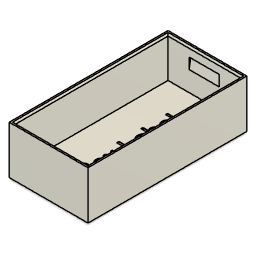
Box Template (Autodesk Fusion 360 design; units mm, degrees)
Autodesk Fusion 360 part; units mm, degrees
sketch "Base" plane through (0, 0, 0) normal (0, 1, 0) x (1, 0, 0)
  line L0 (0, 0) -> (50.8, 0) construction
  line L1 (50.8, 0) -> (50.8, 101.6) construction
  line L2 (50.8, 101.6) -> (0, 101.6) construction
  line L3 (0, 101.6) -> (0, 0) construction
  circle A0 centre (25.4, 25.4) radius 5.9055
  circle A1 centre (25.4, 76.2) radius 5.9055
  line L4 (50.419, 0.381) -> (50.419, 101.219)
  line L5 (50.419, 101.219) -> (0.381, 101.219)
  line L6 (0.381, 101.219) -> (0.381, 0.381)
  line L7 (0.381, 0.381) -> (50.419, 0.381)
  dimension "d1" = 50.8
  dimension "d2" = 101.6
  dimension "d3" = 11.811
  dimension "d5" = 25.4
  dimension "d6" = 25.4
  dimension "d9" = 50.8
  dimension "d10" = 50.8
  constraint horizontal L0
  constraint vertical L1
  constraint horizontal L2
  constraint vertical L3
  constraint coincident L0.start L3.end
  measures "d1" distance of L0.start L0.end
  measures "d2" distance of L0.start L2.end
  measures "d3" diameter of A0
  measures "d5" distance of L0 A0.centre
  measures "d6" distance of L3 A0.centre
extrude "Extrude1" add sketch "Base" along normal blind 6.35 contours A0 | A1 | L4 L5 L6 L7 makes body 1
extrude "Extrude2" cut sketch "Base" along normal blind 5.334 contours A0 bodies 1
chamfer "Chamfer2" distance 1.27 angle 45 1 edges at (19.8941, 0, -23.2645) on bodies 1
pattern_linear "R-Pattern1" count 1 spacing 50.8 along (1, 0, 0) count 2 spacing 50.8 along (0, 0, -1) of "Extrude2", "Chamfer2"
chamfer "Chamfer1" distance 1.27 angle 45 4 edges at (50.419, 0, -50.8) (25.4, 0, -0.381) (0.381, 0, -50.8) (25.4, 0, -101.219) on bodies 1
sketch "Bottom" plane through (0, 6.35, 0) normal (0, 1, 0) x (-1, 0, 0)
  line L0 (-50.419, -101.219) -> (-0.381, -101.219)
  line L1 (-50.419, -0.381) -> (-50.419, -101.219)
  line L2 (-0.381, -0.381) -> (-50.419, -0.381)
  line L3 (-0.381, -101.219) -> (-0.381, -0.381)
  line L4 (-2.413, -2.413) -> (-48.387, -2.413)
  line L5 (-48.387, -2.413) -> (-48.387, -99.187)
  line L6 (-48.387, -99.187) -> (-2.413, -99.187)
  line L7 (-2.413, -99.187) -> (-2.413, -2.413)
  line L8 (-48.387, -2.413) -> (-48.387, -99.187) construction
  line L9 (-48.387, -99.187) -> (-2.413, -99.187) construction
  line L10 (-2.413, -99.187) -> (-2.413, -2.413) construction
  line L11 (-2.413, -2.413) -> (-48.387, -2.413) construction
  dimension "d32" = 2.032
  dimension "d33" = 2.032
  dimension "d34" = 2.032
  dimension "d35" = 2.032
  dimension "d54" = 10.0076
  text T0 "Box Label" font "Arial" height 10.0076 align centre middle in box 96.774 x 45.974 at (-48.387, -2.413) x (0, -1) y (1, 0) spacing 1
  constraint horizontal L6
  constraint horizontal L4
  constraint vertical L5
  constraint vertical L7
  constraint coincident L5.end
  constraint coincident L6.end
  constraint coincident L4.end
  measures "d32" distance of L1 L5
  measures "d33" distance of L3 L7
  measures "d34" distance of L2 L4
  measures "d35" distance of L0 L6
extrude "Extrude3" add sketch "Bottom" along normal blind 25.4 bodies 1
sketch "NotchSize" plane through (0, 0, -99.187) normal (0, 0, 1) x (1, 0, 0)
  line L0 (2.413, 6.35) -> (48.387, 6.35)
  line L1 (48.387, 6.35) -> (48.387, 31.75)
  line L2 (48.387, 31.75) -> (2.413, 31.75)
  line L3 (2.413, 31.75) -> (2.413, 6.35)
  line L4 (2.413, 6.35) -> (2.413, 31.75) construction
  line L5 (2.413, 31.75) -> (48.387, 31.75) construction
  line L6 (48.387, 6.35) -> (48.387, 31.75) construction
  line L7 (15.875, 25.4) -> (34.925, 25.4)
  line L8 (34.925, 25.4) -> (34.925, 19.05)
  line L9 (34.925, 19.05) -> (15.875, 19.05)
  line L10 (15.875, 19.05) -> (15.875, 25.4)
  line L11 (25.4, 25.4) -> (25.4, 31.75) construction
  dimension "d38" = 19.05
  dimension "d39" = 6.35
  dimension "d40" = 6.35
  constraint horizontal L7
  constraint vertical L8
  constraint horizontal L9
  constraint vertical L10
  constraint midpoint L7 L11.start
  constraint midpoint L2 L11.end
  constraint vertical L11
  measures "d38" distance of L7.start L7.end
  measures "d39" distance of L7.start L9.end
  measures "d40" distance of L11.start L11.end
ref_plane "WorkPlane1" through (15.875, 0, 0) normal (1, 0, 0) x (0, 1, 0)
sketch "Notch" plane through (15.875, 0, 0) normal (1, 0, 0) x (0, 0, -1)
  line L0 (99.187, 19.05) -> (99.187, 25.4)
  line L1 (99.187, 25.4) -> (100.203, 25.4)
  line L2 (100.203, 25.4) -> (99.187, 19.05)
  dimension "d42" = 1.016
  constraint coincident L0.end L1.start
  constraint perpendicular L0 L1
  constraint coincident L0.start L2.end
  measures "d42" distance of L0.end L1.end
extrude "Extrude4" cut sketch "Notch" along normal up to surface (19.05 mm away) bodies 1
ref_plane "WorkPlane2" through (25.4, 19.05, -50.8) normal (0, 0, 1) x (1, 0, 0)
mirror "Mirror2" about plane through (25.4, 19.05, -50.8) normal (0, 0, 1) of "Extrude4"
fillet "Fillet1" radius 0.508 1 edges at (25.4, 25.4, -99.187) on bodies 1
fillet "Fillet1" radius 0.508 1 edges at (25.4, 25.4, -2.413) on bodies 1
copy_body "Body->Comp1" bodies 1 removing the originals makes body 2 in component "Box"
chamfer "Chamfer1'" distance 1.016 angle 45 4 edges at (2.413, 31.75, -50.8) (25.4, 31.75, -99.187) (48.387, 31.75, -50.8) (25.4, 31.75, -2.413) on bodies 2 in component "Box"
extrude "Extrude1'" cut sketch "Bottom" against normal blind 0.254 text T0 bodies 2 in component "Box"
component "Box" placed x (1, 0, 0) y (0, 1, 0) z (0, 0, 1) at (0, 0, 0)
equation "d1 = ( 2 * width ) * 1 in"
equation "d2 = ( 2 * length ) * 1 in"
equation "d3 = pegDiameter"
equation "pegDiameter = 0.45 in + 0.015 in"
equation "d7 = width"
equation "d11 = baseHeight"
equation "d13 = pegdepth"
equation "pegdepth = 0.21 in"
equation "baseHeight = 0.25 in"
equation "length = 2"
equation "width = 1"
equation "d22 = width"
equation "d23 = length"
equation "d27 = height - baseHeight"
equation "d29 = -tolerance"
equation "wall = 0.08 in"
equation "d32 = wall"
equation "d33 = wall"
equation "d34 = wall"
equation "d35 = wall"
equation "tolerance = 0.015 in"
equation "height = 1.25 in"
equation "d42 = wall / 2"
equation "d53 = wall / 2"
equation "labelEngrave = 0.01 in"
equation "d56 = -labelEngrave"
named bodies: "Box"
